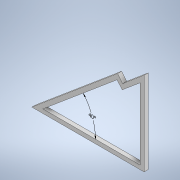
# Autodesk Inventor part: ballRampWithPocketForPowerCell
Saved by Autodesk Inventor 2020.2 (Build 242310000, 310)
## iProperties
Created: 2020-01-25
Part Number: ballRampWithPocketForPowerCell
Material: Generic
Document SubType Name: Modeling
Designer: robst
Density: 1 g/cm^3
Appearance: Default
Author: robst
Autodesk Inventor part; units mm, degrees
sketch "Sketch1" plane through (0, 0, 0) normal (0, 0, 1) x (1, 0, 0)
  line L0 (0, 0) -> (544.8108, 457.1505)
  line L1 (0, 0) -> (749.0326, 0)
  line L2 (713.6671, 532.5231) -> (713.6671, 0)
  line L3 (713.6671, 532.5231) -> (577.4644, 418.2355)
  line L4 (577.4644, 418.2355) -> (544.8108, 457.1505)
  line L5 (69.7859, 25.4) -> (688.2671, 25.4)
  line L6 (688.2671, 25.4) -> (688.2671, 478.0527)
  line L7 (688.2671, 478.0527) -> (574.3337, 382.4512)
  line L8 (574.3337, 382.4512) -> (541.6801, 421.3662)
  line L9 (541.6801, 421.3662) -> (69.7859, 25.4)
  line L10 (688.2671, 511.21) -> (688.2671, 628.3123) construction
  line L11 (69.7859, 25.4) -> (39.5154, 0)
  line L12 (577.4644, 418.2355) -> (593.7912, 398.778) construction
  line L13 (688.2671, 25.4) -> (688.2671, 0) construction
  line L14 (688.2671, 25.4) -> (713.6671, 25.4) construction
  line L15 (541.6801, 421.3662) -> (525.3533, 440.8237) construction
  dimension "d10" = 40
  dimension "d14" = 177.8
  dimension "d15" = 711.2
  dimension "d16" = 50.8
  dimension "d17" = 25.4
  dimension "d18" = 25.4
  dimension "d19" = 25.4
  dimension "d20" = 25.4
  dimension "d21" = 25.4
  dimension "d33" = 50
  dimension "d36" = 76.2
  dimension "d40" = 618.4812
  dimension "d41" = 648.7517
  dimension "d42" = 688.2671
  dimension "d43" = 713.6671
  dimension "d44" = 452.6526
  dimension "d45" = 478.0527
  dimension "d46" = 507.1231
  dimension "d47" = 532.5231
  dimension "d48" = 685.8
  constraints: 32 end point, 9 perpendicular, 7 point on line, 3 parallel, 2 horizontal, 1 vertical
  measures "d10" angle of L0 L1
  measures "d14" distance of L2.start L3.end
  measures "d15" distance of L0.start L0.end
  measures "d16" distance of L3.end L0.end
  measures "d17" distance between parallel lines of L5 L1
  measures "d18" distance between parallel lines of L6 L2
  measures "d19" distance between parallel lines of L0 L9
  measures "d20" distance between parallel lines of L8 L4
  measures "d21" distance between parallel lines of L3 L7
  measures "d33" angle of L6 L7
  measures "d36" distance between parallel lines of L7 L0
  measures "d40" distance of L5.end L5.start
  measures "d41" distance of L13.end L11.end
  measures "d42" horizontal distance of L5.end L0.start
  measures "d43" distance of L2.end L0.start
  measures "d44" distance of L6.end L5.end
  measures "d45" distance of L13.end L6.end
  measures "d46" distance of L14.end L2.start
  measures "d47" distance of L2.end L2.start
  measures "d48" distance from line of L15 L0.start
extrude "Extrusion1" add sketch "Sketch1" along normal mid plane 25.4
ref_plane "planeForPowerCells" through (-48.9804, 58.3726, 12.7) normal (-0.6428, 0.766, 0) x (0.766, 0.6428, 0)
ref_plane "planeForShootingPowerCells" through (528.484, 476.6081, 12.7) normal (-0.6428, 0.766, 0) x (0.766, 0.6428, 0)
ref_plane "Work Plane3" through (612.9122, 514.2944, 12.7) normal (0.766, 0.6428, 0) x (0, 0, -1)
body "Solid1"
